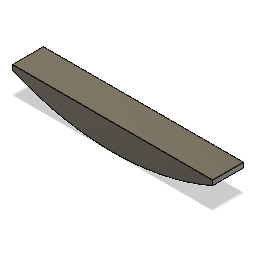
Wedge (Autodesk Fusion 360 design; units mm, degrees)
Autodesk Fusion 360 part; units mm, degrees
sketch "Sketch1" plane through (0, 0, 0) normal (0, 0, 1) x (1, 0, 0)
  arc A0 (-40, 0) -> (-36, 0) centre (-38, 4.5826) ccw
  line L0 (-38, 6.5) -> (-38, 5)
  line L1 (-40, 0) -> (-40, 0.1)
  line L2 (-40, 0.1) -> (-36, 0.1)
  line L3 (-36, 0.1) -> (-36, 0)
  dimension "d2" = 5
  measures "d2" radius of A0
extrude "Extrude1" add sketch "Sketch1" along normal blind 0.62
sketch "Sketch2" plane through (-40, 0, 0) normal (-1, 0, 0) x (0, 0, 1)
  line L0 (0, 0.1) -> (0, 0)
  line L1 (0, 0) -> (0.62, 0)
  line L2 (0.62, 0) -> (0.62, 0.1)
  line L3 (0.62, 0.1) -> (0, 0.1)
sketch "Sketch3" plane through (0, 0.1, 0) normal (0, 1, 0) x (-1, 0, 0)
  line L0 (36, 0) -> (40, 0)
  line L1 (40, 0) -> (40, 0.62)
  line L2 (40, 0.62) -> (36, 0.62)
  line L3 (36, 0.62) -> (36, 0)
